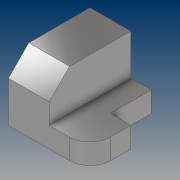
# Autodesk Inventor part: 47
Saved by Autodesk Inventor 2020.2 (Build 242310000, 310)
## iProperties
Created: 2020-09-17
Part Number: 47
Material: 鋼、碳鋼
Document SubType Name: Modeling
Designer: user
Density: 7.85 g/cm^3
Appearance: 半拋光
Mass: 225.965 g
Surface Area: 64.97 cm^2
Volume: 28.7854 cm^3
Author: user
Autodesk Inventor part; units mm, degrees
ref_plane "YZ Plane" through (0, 0, 0) normal (1, 0, 0) x (0, 1, 0)
ref_plane "XZ Plane" through (0, 0, 0) normal (0, 1, 0) x (-1, 0, 0)
ref_plane "XY Plane" through (0, 0, 0) normal (0, 0, 1) x (1, 0, 0)
sketch "草圖1" plane through (0, 0, 0) normal (0, 1, 0) x (-1, 0, 0)
  line L0 (0, 0) -> (-40, 0)
  line L1 (-40, 0) -> (-40, 40)
  line L2 (-40, 40) -> (0, 40)
  line L3 (0, 40) -> (0, 0)
  line L4 (-40, 0) -> (-30, 0)
  line L5 (-30, 0) -> (-30, 20)
  line L6 (-30, 20) -> (-40, 20)
  line L7 (-40, 20) -> (-40, 0)
  dimension "d0" = 40
  dimension "d1" = 40
  dimension "d2" = 10
  dimension "d3" = 20
  constraints: 16 end point, 4 parallel, 2 horizontal, 2 perpendicular
  measures "d0" distance of L2.end L0.start
  measures "d1" distance of L1.end L2.end
  measures "d2" distance of L5.end L6.end
  measures "d3" distance of L4.end L5.end
extrude "擠出1" add sketch "草圖1" along normal blind 10 contours L0 L5 L6 L1 L2 L3
sketch "草圖2" plane through (0, 10, 0) normal (0, 1, 0) x (1, 0, 0)
  line L0 (30, 0) -> (30, -20) projected
  line L1 (30, -20) -> (40, -20) projected
  line L2 (40, -20) -> (40, -40) projected
  line L3 (40, -40) -> (0, -40) projected
  line L4 (0, -40) -> (0, 0) projected
  line L5 (0, 0) -> (30, 0) projected
  line L6 (0, -40) -> (20, -40)
  line L7 (20, -40) -> (20, 0)
  line L8 (20, 0) -> (0, 0)
  line L9 (0, 0) -> (0, -40)
  line L10 (30, 0) -> (0, 0) projected
  point P0 (20, 0)
  dimension "d6" = 20
  constraints: 8 end point, 2 parallel, 1 collinear, 1 horizontal, 1 perpendicular
  measures "d6" distance between parallel lines of L4 L7
extrude "擠出2" add sketch "草圖2" along normal blind 20 contours L7 L3 L4 L5
chamfer "倒角1" distance 10 angle 45 1 edges at (10, 30, 40)
fillet "圓角1" radius 10 1 edges at (40, 5, 40)
